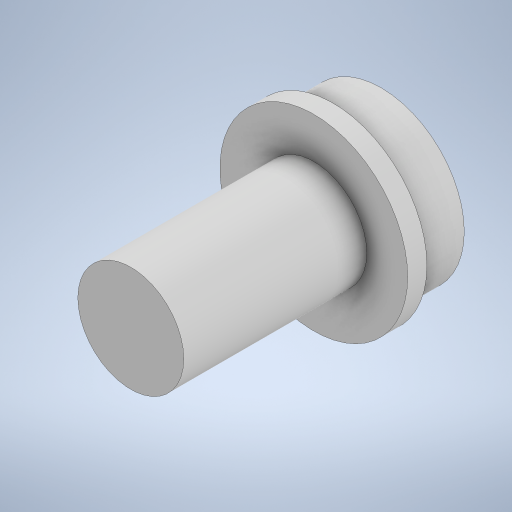
# Autodesk Inventor part: деталь ек
Saved by Autodesk Inventor 2024.2 (Build 282272000, 272)
## iProperties
Created: 2025-12-06
Part Number: деталь ек
Material: Типовые
Document SubType Name: Modeling
Designer: Zakhar
Density: 1 g/cm^3
Appearance: По умолчанию
Author: Zakhar
Autodesk Inventor part; units mm, degrees
ref_plane "YZ Plane" through (0, 0, 0) normal (1, 0, 0) x (0, 1, 0)
ref_plane "XZ Plane" through (0, 0, 0) normal (0, 1, 0) x (-1, 0, 0)
ref_plane "XY Plane" through (0, 0, 0) normal (0, 0, 1) x (1, 0, 0)
sketch "Эскиз1" plane through (0, 0, 0) normal (0, 0, 1) x (1, 0, 0)
  circle A0 centre (0, 0) radius 8.625
  circle A1 centre (0, 0) radius 9.75
  circle A2 centre (0, 0) radius 5.5
  dimension "d0" = 17.25
  dimension "d1" = 19.5
  dimension "d2" = 11
  constraints: 3 centre point, 3 coincident
  measures "d0" diameter of A0
  measures "d1" diameter of A1
  measures "d2" diameter of A2
extrude "Выдавливание1" add sketch "Эскиз1" along normal blind 19 contours A2
extrude "Выдавливание2" add sketch "Эскиз1" against normal blind 2 contours A0 | A1 | A2
extrude "Выдавливание3" add sketch "Эскиз1" against normal blind 7 contours A0 | A2
